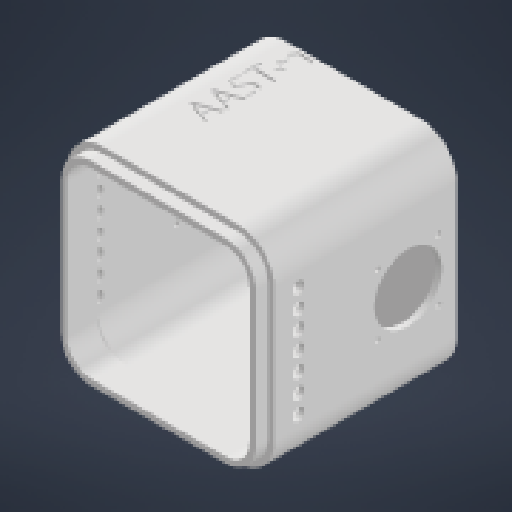
# Autodesk Inventor part: bottom case
Saved by Autodesk Inventor 2024 (Build 280153000, 153)
## iProperties
Created: 2023-06-18
Part Number: bottom case
Material: 일반
Document SubType Name: Modeling
Designer: 6gioc
Density: 1 g/cm^3
Appearance: 기본값
Author: 6gioc
Autodesk Inventor part; units mm, degrees
ref_plane "YZ Plane" through (0, 0, 0) normal (1, 0, 0) x (0, 1, 0)
ref_plane "XZ Plane" through (0, 0, 0) normal (0, 1, 0) x (-1, 0, 0)
ref_plane "XY Plane" through (0, 0, 0) normal (0, 0, 1) x (1, 0, 0)
sketch "스케치1" plane through (0, 0, 0) normal (0, 0, 1) x (1, 0, 0)
  line L0 (-30, 0) -> (-140, 0)
  line L1 (-170, -30) -> (-170, -140)
  line L2 (-140, -170) -> (-30, -170)
  line L3 (0, -140) -> (0, -30)
  arc A0 (-30, -170) -> (0, -140) centre (-30, -140) ccw
  arc A1 (-170, -140) -> (-140, -170) centre (-140, -140) ccw
  arc A2 (-140, 0) -> (-170, -30) centre (-140, -30) ccw
  arc A3 (0, -30) -> (-30, 0) centre (-30, -30) ccw
  point P0 (0, 0)
  point P1 (-170, -170)
  point P2 (-170, 0)
  point P3 (0, -170)
  dimension "d0" = 170
  dimension "d1" = 170
  dimension "d2" = 30
  dimension "d3" = 30
  dimension "d4" = 30
  constraints: 8 end point, 8 point on circle, 8 point on line, 8 tangent, 4 centre point, 2 parallel, 1 equal radius, 1 horizontal, 1 perpendicular
  measures "d0" distance of point (0, -170) point (-170, -170)
  measures "d1" distance of point (-170, -170) point (-170, 0)
  measures "d2" radius of A0
  measures "d3" radius of A1
  measures "d4" radius of A3
extrude "돌출1" add sketch "스케치1" along normal blind 150
shell "쉘1" thickness 5 removed faces 1 at (-66.6667, -113.3333, 150)
sketch "스케치2" plane through (0, 0, 150) normal (0, 0, 1) x (1, 0, 0)
  line L0 (-30, 0) -> (-140, 0)
  line L1 (-170, -30) -> (-170, -140)
  line L2 (-140, -170) -> (-30, -170)
  line L3 (0, -140) -> (0, -30)
  arc A0 (-30, -170) -> (0, -140) centre (-30, -140) ccw
  arc A1 (0, -30) -> (-30, 0) centre (-30, -30) ccw
  arc A2 (-140, 0) -> (-170, -30) centre (-140, -30) ccw
  arc A3 (-170, -140) -> (-140, -170) centre (-140, -140) ccw
  line L4 (-160, -30) -> (-160, -140)
  arc A4 (-160, -140) -> (-140, -160) centre (-140, -140) ccw
  line L5 (-140, -160) -> (-30, -160)
  arc A5 (-30, -160) -> (-10, -140) centre (-30, -140) ccw
  line L6 (-10, -140) -> (-10, -30)
  arc A6 (-10, -30) -> (-30, -10) centre (-30, -30) ccw
  line L7 (-30, -10) -> (-140, -10)
  arc A7 (-140, -10) -> (-160, -30) centre (-140, -30) ccw
  line L8 (-5, -140) -> (-5, -30)
  arc A8 (-5, -30) -> (-30, -5) centre (-30, -30) ccw
  line L9 (-30, -5) -> (-140, -5)
  arc A9 (-140, -5) -> (-165, -30) centre (-140, -30) ccw
  line L10 (-165, -30) -> (-165, -140)
  arc A10 (-165, -140) -> (-140, -165) centre (-140, -140) ccw
  line L11 (-140, -165) -> (-30, -165)
  arc A11 (-30, -165) -> (-5, -140) centre (-30, -140) ccw
  point P0 (0, 0)
  point P1 (-170, -170)
  point P2 (-170, 0)
  point P3 (0, -170)
  dimension "d8" = 170
  dimension "d9" = 170
  dimension "d10" = 30
  dimension "d11" = 10
  dimension "d17" = 5
  constraints: 24 end point, 24 point on circle, 12 centre point, 8 point on line, 8 tangent, 6 parallel, 3 equal radius, 3 perpendicular, 1 horizontal, 14 other
  measures "d8" distance of point (0, -170) point (-170, -170)
  measures "d9" distance of point (-170, -170) point (-170, 0)
  measures "d10" radius of A0
  measures "d11" radial gap between concentric circles of A2 A7
  measures "d17" radial gap between concentric circles of A0 A11
extrude "돌출2" add sketch "스케치2" against normal blind 20 contours A1 L3 A0 L2 A3 L1 A2 L0 | A11 L11 A10 L10 A9 L9 A8 L8
chamfer "모따기1" distance 5 angle 45 8 edges at (-85, -160, 130) (-15.8579, -154.1421, 130) (-10, -85, 130) (-15.8579, -15.8579, 130) (-85, -10, 130) (-154.1421, -15.8579, 130) (-160, -85, 130) (-154.1421, -154.1421, 130)
extrude "돌출3" add sketch "스케치2" along normal blind 10 contours A11 L11 A10 L10 A9 L9 A8 L8
sketch "스케치3" plane through (-140, 0, 0) normal (0, 1, 0) x (1, 0, 0)
  line L0 (23.785, -91.5699) -> (3.785, -84.2336)
  line L1 (3.785, -84.2336) -> (3.785, -81.9279)
  line L2 (3.785, -81.9279) -> (23.785, -74.6266)
  line L3 (23.785, -74.6266) -> (23.785, -77.107)
  line L4 (23.785, -77.107) -> (17.9509, -79.2205)
  line L5 (17.9509, -79.2205) -> (17.9509, -87.238)
  line L6 (17.9509, -87.238) -> (23.785, -89.2991)
  line L7 (23.785, -89.2991) -> (23.785, -91.5699)
  line L8 (6.9465, -83.2729) -> (15.9422, -86.5568)
  line L9 (15.9422, -86.5568) -> (15.9422, -79.9716)
  line L10 (15.9422, -79.9716) -> (6.9465, -83.2205)
  line L11 (6.9465, -83.2205) -> (6.9465, -83.2729)
  line L12 (23.785, -73.5262) -> (3.785, -66.1899)
  line L13 (3.785, -66.1899) -> (3.785, -63.8843)
  line L14 (3.785, -63.8843) -> (23.785, -56.583)
  line L15 (23.785, -56.583) -> (23.785, -59.0633)
  line L16 (23.785, -59.0633) -> (17.9509, -61.1768)
  line L17 (17.9509, -61.1768) -> (17.9509, -69.1943)
  line L18 (17.9509, -69.1943) -> (23.785, -71.2555)
  line L19 (23.785, -71.2555) -> (23.785, -73.5262)
  line L20 (6.9465, -65.2292) -> (15.9422, -68.5131)
  line L21 (15.9422, -68.5131) -> (15.9422, -61.9279)
  line L22 (15.9422, -61.9279) -> (6.9465, -65.1768)
  line L23 (6.9465, -65.1768) -> (6.9465, -65.2292)
  spline S0 degree 2 poles (24.1518, -49.1768) (24.1518, -52.4607) (22.8068, -54.8712) knots 0 0 0 1 1 1
  line L24 (22.8068, -54.8712) -> (20.8155, -54.8712)
  spline S1 degree 2 poles (20.8155, -54.8712) (22.1256, -52.321) (22.1256, -49.2817) knots 0 0 0 1 1 1
  spline S2 degree 2 poles (22.1256, -49.2817) (22.1256, -47.0284) (20.2042, -44.8624) (18.5098, -44.8624) knots 0 0 0 1 2 2 2
  spline S3 degree 2 poles (18.5098, -44.8624) (17.0251, -44.8624) (15.4356, -46.3821) (14.8417, -48.2511) knots 0 0 0 1 2 2 2
  line L25 (14.8417, -48.2511) -> (14.1605, -50.1899)
  spline S4 degree 2 poles (14.1605, -50.1899) (13.4094, -52.4083) (10.9465, -54.5742) (8.7631, -54.5742) knots 0 0 0 1 2 2 2
  spline S5 degree 2 poles (8.7631, -54.5742) (6.3526, -54.5742) (3.4531, -51.3952) (3.4531, -48.3559) knots 0 0 0 1 2 2 2
  spline S6 degree 2 poles (3.4531, -48.3559) (3.4531, -45.7533) (4.5535, -43.4825) knots 0 0 0 1 1 1
  line L26 (4.5535, -43.4825) -> (6.5622, -43.4825)
  spline S7 degree 2 poles (6.5622, -43.4825) (5.4443, -45.8755) (5.4443, -48.4432) knots 0 0 0 1 1 1
  spline S8 degree 2 poles (5.4443, -48.4432) (5.4443, -50.2598) (7.1212, -52.2511) (9.9858, -52.2511) (11.4705, -50.976) (12.0644, -49.2817) knots 0 0 0 1 2 3 4 4 4
  line L27 (12.0644, -49.2817) -> (12.6932, -47.3079)
  spline S9 degree 2 poles (12.6932, -47.3079) (13.5317, -44.8275) (15.9771, -42.4694) (18.3352, -42.4694) knots 0 0 0 1 2 2 2
  spline S10 degree 2 poles (18.3352, -42.4694) (21.0426, -42.4694) (24.1518, -45.7882) (24.1518, -49.1768) knots 0 0 0 1 2 2 2
  line L28 (23.785, -34.0677) -> (5.7762, -34.0677)
  line L29 (5.7762, -34.0677) -> (5.7762, -40.1812)
  line L30 (5.7762, -40.1812) -> (3.785, -40.1812)
  line L31 (3.785, -40.1812) -> (3.785, -25.631)
  line L32 (3.785, -25.631) -> (5.7762, -25.631)
  line L33 (5.7762, -25.631) -> (5.7762, -31.7445)
  line L34 (5.7762, -31.7445) -> (23.785, -31.7445)
  line L35 (23.785, -31.7445) -> (23.785, -34.0677)
  spline S11 degree 2 poles (9.9173, -17.3252) (11.1446, -16.9103) (12.5448, -14.4038) (12.5448, -13.1592) knots 0 0 0 1 2 2 2
  spline S12 degree 2 poles (12.5448, -13.1592) (12.5448, -11.6208) (10.9199, -8.9587) (9.416, -8.5438) knots 0 0 0 1 2 2 2
  spline S13 degree 2 poles (9.416, -8.5438) (9.8481, -6.7979) (11.8706, -3.7037) (12.804, -3.0469) knots 0 0 0 1 2 2 2
  spline S14 degree 2 poles (12.804, -3.0469) (13.8585, -2.3208) (15.2068, -2.3208) knots 0 0 0 1 1 1
  spline S15 degree 2 poles (15.2068, -2.3208) (16.123, -2.3208) (17.2811, -2.7703) knots 0 0 0 1 1 1
  spline S16 degree 2 poles (17.2811, -2.7703) (18.1973, -3.2197) (18.8369, -3.2197) knots 0 0 0 1 1 1
  spline S17 degree 2 poles (18.8369, -3.2197) (19.3036, -3.2197) (20.8594, -2.5801) knots 0 0 0 1 1 1
  spline S18 degree 2 poles (20.8594, -2.5801) (21.8447, -2.2863) (22.3114, -2.2863) knots 0 0 0 1 1 1
  spline S19 degree 2 poles (22.3114, -2.2863) (23.6943, -2.2863) (25.1117, -3.4617) knots 0 0 0 1 1 1
  spline S20 degree 2 poles (25.1117, -3.4617) (27.0651, -5.2422) (29.2258, -10.3243) (29.2258, -13.1074) knots 0 0 0 1 2 2 2
  spline S21 degree 2 poles (29.2258, -13.1074) (29.2258, -16.0114) (25.8378, -20.4367) (23.2103, -20.4367) knots 0 0 0 1 2 2 2
  spline S22 degree 2 poles (23.2103, -20.4367) (21.7755, -20.4367) (20.5482, -19.8144) knots 0 0 0 1 1 1
  spline S23 degree 2 poles (20.5482, -19.8144) (19.7185, -19.2958) (18.8715, -19.2958) knots 0 0 0 1 1 1
  spline S24 degree 2 poles (18.8715, -19.2958) (18.059, -19.2958) (17.2811, -19.6242) knots 0 0 0 1 1 1
  spline S25 degree 2 poles (17.2811, -19.6242) (15.2241, -20.4367) (14.4981, -20.4367) knots 0 0 0 1 1 1
  spline S26 degree 2 poles (14.4981, -20.4367) (12.5102, -20.4367) (11.0063, -19.0883) knots 0 0 0 1 1 1
  spline S27 degree 2 poles (11.0063, -19.0883) (10.384, -18.466) (9.9173, -17.3252) knots 0 0 0 1 1 1
  spline S28 degree 2 poles (19.7531, -19.6934) (19.7531, -21.8023) (18.3183, -23.5654) knots 0 0 0 1 1 1
  spline S29 degree 2 poles (18.3183, -23.5654) (16.97, -25.0348) (14.5672, -25.3805) knots 0 0 0 1 1 1
  spline S30 degree 2 poles (14.5672, -25.3805) (14.5672, -22.9604) (15.9328, -21.3528) knots 0 0 0 1 1 1
  spline S31 degree 2 poles (15.9328, -21.3528) (17.454, -19.6934) (19.7531, -19.6934) knots 0 0 0 1 1 1
  point P0 (140, 0)
  point P1 (3.4531, -92.1288)
  constraints: 1 other
extrude "돌출4" cut sketch "스케치3" against normal blind 2
sketch "스케치4" plane through (-140, -170, 0) normal (0, -1, 0) x (1, 0, 0)
  line L0 (-0.2518, 7.0228) -> (110.1783, 7.0228) construction
  line L1 (110.1783, 7.0228) -> (110.1783, 29.5331) construction
  line L2 (110.1783, 29.5331) -> (-0.2518, 29.5331) construction
  line L3 (-0.2518, 29.5331) -> (-0.2518, 7.0228) construction
  line L4 (82.8987, 6.8718) -> (109.9483, 6.8718) construction
  line L5 (109.9483, 6.8718) -> (109.9483, 3.7565) construction
  line L6 (109.9483, 3.7565) -> (82.8987, 3.7565) construction
  line L7 (82.8987, 3.7565) -> (82.8987, 6.8718) construction
  line L8 (6.2831, 27.4497) -> (5.0902, 27.4497)
  line L9 (5.0902, 27.4497) -> (1.5505, 34.3476)
  line L10 (1.5505, 34.3476) -> (1.5505, 27.4497)
  line L11 (1.5505, 27.4497) -> (0.5586, 27.4497)
  line L12 (0.5586, 27.4497) -> (0.5586, 35.4497)
  line L13 (0.5586, 35.4497) -> (2.0692, 35.4497)
  line L14 (2.0692, 35.4497) -> (5.2912, 29.1159)
  line L15 (5.2912, 29.1159) -> (5.2912, 35.4497)
  line L16 (5.2912, 35.4497) -> (6.2831, 35.4497)
  line L17 (6.2831, 35.4497) -> (6.2831, 27.4497)
  spline S0 degree 2 poles (13.5635, 34.5356) (14.0173, 34.004) (14.523, 32.4481) (14.523, 31.4497) knots 0 0 0 1 2 2 2
  spline S1 degree 2 poles (14.523, 31.4497) (14.523, 30.4773) (14.0303, 28.9019) (13.5635, 28.3703) knots 0 0 0 1 2 2 2
  spline S2 degree 2 poles (13.5635, 28.3703) (13.0708, 27.8128) (11.7677, 27.2812) (10.9833, 27.2812) knots 0 0 0 1 2 2 2
  spline S3 degree 2 poles (10.9833, 27.2812) (10.1729, 27.2812) (8.8763, 27.8322) (8.403, 28.3703) knots 0 0 0 1 2 2 2
  spline S4 degree 2 poles (8.403, 28.3703) (7.9427, 28.9019) (7.45, 30.4643) (7.45, 31.4497) knots 0 0 0 1 2 2 2
  spline S5 degree 2 poles (7.45, 31.4497) (7.45, 32.4546) (7.9492, 33.9846) (8.4095, 34.5356) knots 0 0 0 1 2 2 2
  spline S6 degree 2 poles (8.4095, 34.5356) (8.8763, 35.0672) (10.1794, 35.6183) (10.9833, 35.6183) knots 0 0 0 1 2 2 2
  spline S7 degree 2 poles (10.9833, 35.6183) (11.8001, 35.6183) (13.1097, 35.0478) (13.5635, 34.5356) knots 0 0 0 1 2 2 2
  spline S8 degree 2 poles (13.4144, 31.4497) (13.4144, 32.2407) (13.0708, 33.4659) (12.7596, 33.8679) knots 0 0 0 1 2 2 2
  spline S9 degree 2 poles (12.7596, 33.8679) (12.4419, 34.2828) (11.5473, 34.6977) (10.9897, 34.6977) knots 0 0 0 1 2 2 2
  spline S10 degree 2 poles (10.9897, 34.6977) (10.4128, 34.6977) (9.544, 34.2958) (9.2134, 33.8679) knots 0 0 0 1 2 2 2
  spline S11 degree 2 poles (9.2134, 33.8679) (8.8957, 33.4595) (8.5586, 32.2277) (8.5586, 31.4497) knots 0 0 0 1 2 2 2
  spline S12 degree 2 poles (8.5586, 31.4497) (8.5586, 29.8744) (9.8811, 28.2018) (10.9897, 28.2018) knots 0 0 0 1 2 2 2
  spline S13 degree 2 poles (10.9897, 28.2018) (12.0983, 28.2018) (13.4144, 29.8744) (13.4144, 31.4497) knots 0 0 0 1 2 2 2
  line L18 (17.557, 27.4497) -> (17.557, 34.5032)
  line L19 (17.557, 34.5032) -> (14.873, 34.5032)
  line L20 (14.873, 34.5032) -> (14.873, 35.4497)
  line L21 (14.873, 35.4497) -> (21.3042, 35.4497)
  line L22 (21.3042, 35.4497) -> (21.3042, 34.5032)
  line L23 (21.3042, 34.5032) -> (18.6202, 34.5032)
  line L24 (18.6202, 34.5032) -> (18.6202, 27.4497)
  line L25 (18.6202, 27.4497) -> (17.557, 27.4497)
  line L26 (30.335, 34.5032) -> (26.6137, 34.5032)
  line L27 (26.6137, 34.5032) -> (26.6137, 32.2471)
  line L28 (26.6137, 32.2471) -> (30.1794, 32.2471)
  line L29 (30.1794, 32.2471) -> (30.1794, 31.3006)
  line L30 (30.1794, 31.3006) -> (26.6137, 31.3006)
  line L31 (26.6137, 31.3006) -> (26.6137, 27.4497)
  line L32 (26.6137, 27.4497) -> (25.5505, 27.4497)
  line L33 (25.5505, 27.4497) -> (25.5505, 35.4497)
  line L34 (25.5505, 35.4497) -> (30.335, 35.4497)
  line L35 (30.335, 35.4497) -> (30.335, 34.5032)
  spline S14 degree 2 poles (36.9476, 34.5356) (37.4014, 34.004) (37.9071, 32.4481) (37.9071, 31.4497) knots 0 0 0 1 2 2 2
  spline S15 degree 2 poles (37.9071, 31.4497) (37.9071, 30.4773) (37.4144, 28.9019) (36.9476, 28.3703) knots 0 0 0 1 2 2 2
  spline S16 degree 2 poles (36.9476, 28.3703) (36.4549, 27.8128) (35.1518, 27.2812) (34.3674, 27.2812) knots 0 0 0 1 2 2 2
  spline S17 degree 2 poles (34.3674, 27.2812) (33.557, 27.2812) (32.2604, 27.8322) (31.7871, 28.3703) knots 0 0 0 1 2 2 2
  spline S18 degree 2 poles (31.7871, 28.3703) (31.3269, 28.9019) (30.8341, 30.4643) (30.8341, 31.4497) knots 0 0 0 1 2 2 2
  spline S19 degree 2 poles (30.8341, 31.4497) (30.8341, 32.4546) (31.3333, 33.9846) (31.7936, 34.5356) knots 0 0 0 1 2 2 2
  spline S20 degree 2 poles (31.7936, 34.5356) (32.2604, 35.0672) (33.5635, 35.6183) (34.3674, 35.6183) knots 0 0 0 1 2 2 2
  spline S21 degree 2 poles (34.3674, 35.6183) (35.1842, 35.6183) (36.4938, 35.0478) (36.9476, 34.5356) knots 0 0 0 1 2 2 2
  spline S22 degree 2 poles (36.7985, 31.4497) (36.7985, 32.2407) (36.4549, 33.4659) (36.1437, 33.8679) knots 0 0 0 1 2 2 2
  spline S23 degree 2 poles (36.1437, 33.8679) (35.826, 34.2828) (34.9314, 34.6977) (34.3739, 34.6977) knots 0 0 0 1 2 2 2
  spline S24 degree 2 poles (34.3739, 34.6977) (33.7969, 34.6977) (32.9281, 34.2958) (32.5975, 33.8679) knots 0 0 0 1 2 2 2
  spline S25 degree 2 poles (32.5975, 33.8679) (32.2799, 33.4595) (31.9427, 32.2277) (31.9427, 31.4497) knots 0 0 0 1 2 2 2
  spline S26 degree 2 poles (31.9427, 31.4497) (31.9427, 29.8744) (33.2653, 28.2018) (34.3739, 28.2018) knots 0 0 0 1 2 2 2
  spline S27 degree 2 poles (34.3739, 28.2018) (35.4824, 28.2018) (36.7985, 29.8744) (36.7985, 31.4497) knots 0 0 0 1 2 2 2
  line L36 (45.2653, 27.4497) -> (43.8844, 27.4497)
  line L37 (43.8844, 27.4497) -> (41.356, 30.6329)
  line L38 (41.356, 30.6329) -> (40.1372, 30.6329)
  line L39 (40.1372, 30.6329) -> (40.1372, 27.4497)
  line L40 (40.1372, 27.4497) -> (39.074, 27.4497)
  line L41 (39.074, 27.4497) -> (39.074, 35.4497)
  line L42 (39.074, 35.4497) -> (41.1356, 35.4497)
  spline S28 degree 2 poles (41.1356, 35.4497) (41.8228, 35.4497) (42.7499, 35.3006) (43.1713, 35.0283) knots 0 0 0 1 2 2 2
  spline S29 degree 2 poles (43.1713, 35.0283) (43.5927, 34.756) (44.0789, 33.9068) (44.0789, 33.2779) knots 0 0 0 1 2 2 2
  spline S30 degree 2 poles (44.0789, 33.2779) (44.0789, 32.4027) (43.1842, 31.2163) (42.4192, 30.9311) knots 0 0 0 1 2 2 2
  line L43 (42.4192, 30.9311) -> (45.2653, 27.4497)
  spline S31 degree 2 poles (42.9703, 33.1937) (42.9703, 33.5437) (42.7239, 34.0818) (42.4646, 34.2569) knots 0 0 0 1 2 2 2
  spline S32 degree 2 poles (42.4646, 34.2569) (42.2377, 34.406) (41.6348, 34.5291) (41.194, 34.5291) knots 0 0 0 1 2 2 2
  line L44 (41.194, 34.5291) -> (40.1372, 34.5291)
  line L45 (40.1372, 34.5291) -> (40.1372, 31.521)
  line L46 (40.1372, 31.521) -> (41.0708, 31.521)
  spline S33 degree 2 poles (41.0708, 31.521) (41.5311, 31.521) (42.2636, 31.6831) (42.5165, 31.936) knots 0 0 0 1 2 2 2
  spline S34 degree 2 poles (42.5165, 31.936) (42.7499, 32.1564) (42.9703, 32.7787) (42.9703, 33.1937) knots 0 0 0 1 2 2 2
  line L47 (7.4176, 14.2779) -> (6.3544, 14.2779)
  line L48 (6.3544, 14.2779) -> (6.3544, 21.1694)
  line L49 (6.3544, 21.1694) -> (4.2669, 16.4822)
  line L50 (4.2669, 16.4822) -> (3.6186, 16.4822)
  line L51 (3.6186, 16.4822) -> (1.5505, 21.1694)
  line L52 (1.5505, 21.1694) -> (1.5505, 14.2779)
  line L53 (1.5505, 14.2779) -> (0.5586, 14.2779)
  line L54 (0.5586, 14.2779) -> (0.5586, 22.2779)
  line L55 (0.5586, 22.2779) -> (2.0108, 22.2779)
  line L56 (2.0108, 22.2779) -> (4.0076, 17.8241)
  line L57 (4.0076, 17.8241) -> (5.9395, 22.2779)
  line L58 (5.9395, 22.2779) -> (7.4176, 22.2779)
  line L59 (7.4176, 22.2779) -> (7.4176, 14.2779)
  line L60 (11.826, 14.2779) -> (8.7272, 14.2779)
  line L61 (8.7272, 14.2779) -> (8.7272, 15.0948)
  line L62 (8.7272, 15.0948) -> (9.745, 15.0948)
  line L63 (9.745, 15.0948) -> (9.745, 21.4611)
  line L64 (9.745, 21.4611) -> (8.7272, 21.4611)
  line L65 (8.7272, 21.4611) -> (8.7272, 22.2779)
  line L66 (8.7272, 22.2779) -> (11.826, 22.2779)
  line L67 (11.826, 22.2779) -> (11.826, 21.4611)
  line L68 (11.826, 21.4611) -> (10.8082, 21.4611)
  line L69 (10.8082, 21.4611) -> (10.8082, 15.0948)
  line L70 (10.8082, 15.0948) -> (11.826, 15.0948)
  line L71 (11.826, 15.0948) -> (11.826, 14.2779)
  line L72 (17.7774, 14.2779) -> (13.1421, 14.2779)
  line L73 (13.1421, 14.2779) -> (13.1421, 22.2779)
  line L74 (13.1421, 22.2779) -> (14.2053, 22.2779)
  line L75 (14.2053, 22.2779) -> (14.2053, 15.2245)
  line L76 (14.2053, 15.2245) -> (17.7774, 15.2245)
  line L77 (17.7774, 15.2245) -> (17.7774, 14.2779)
  line L78 (21.4014, 14.2779) -> (18.3025, 14.2779)
  line L79 (18.3025, 14.2779) -> (18.3025, 15.0948)
  line L80 (18.3025, 15.0948) -> (19.3204, 15.0948)
  line L81 (19.3204, 15.0948) -> (19.3204, 21.4611)
  line L82 (19.3204, 21.4611) -> (18.3025, 21.4611)
  line L83 (18.3025, 21.4611) -> (18.3025, 22.2779)
  line L84 (18.3025, 22.2779) -> (21.4014, 22.2779)
  line L85 (21.4014, 22.2779) -> (21.4014, 21.4611)
  line L86 (21.4014, 21.4611) -> (20.3836, 21.4611)
  line L87 (20.3836, 21.4611) -> (20.3836, 15.0948)
  line L88 (20.3836, 15.0948) -> (21.4014, 15.0948)
  line L89 (21.4014, 15.0948) -> (21.4014, 14.2779)
  line L90 (24.5846, 14.2779) -> (24.5846, 21.3314)
  line L91 (24.5846, 21.3314) -> (21.9006, 21.3314)
  line L92 (21.9006, 21.3314) -> (21.9006, 22.2779)
  line L93 (21.9006, 22.2779) -> (28.3317, 22.2779)
  line L94 (28.3317, 22.2779) -> (28.3317, 21.3314)
  line L95 (28.3317, 21.3314) -> (25.6478, 21.3314)
  line L96 (25.6478, 21.3314) -> (25.6478, 14.2779)
  line L97 (25.6478, 14.2779) -> (24.5846, 14.2779)
  line L98 (28.2799, 14.2779) -> (30.9768, 22.2779)
  line L99 (30.9768, 22.2779) -> (32.2863, 22.2779)
  line L100 (32.2863, 22.2779) -> (34.9833, 14.2779)
  line L101 (34.9833, 14.2779) -> (33.8617, 14.2779)
  line L102 (33.8617, 14.2779) -> (33.1356, 16.5146)
  line L103 (33.1356, 16.5146) -> (30.0821, 16.5146)
  line L104 (30.0821, 16.5146) -> (29.356, 14.2779)
  line L105 (29.356, 14.2779) -> (28.2799, 14.2779)
  line L106 (32.8439, 17.4222) -> (31.6056, 21.1888)
  line L107 (31.6056, 21.1888) -> (30.3739, 17.4222)
  line L108 (30.3739, 17.4222) -> (32.8439, 17.4222)
  line L109 (41.933, 14.2779) -> (40.5521, 14.2779)
  line L110 (40.5521, 14.2779) -> (38.0238, 17.4611)
  line L111 (38.0238, 17.4611) -> (36.805, 17.4611)
  line L112 (36.805, 17.4611) -> (36.805, 14.2779)
  line L113 (36.805, 14.2779) -> (35.7418, 14.2779)
  line L114 (35.7418, 14.2779) -> (35.7418, 22.2779)
  line L115 (35.7418, 22.2779) -> (37.8034, 22.2779)
  spline S35 degree 2 poles (37.8034, 22.2779) (38.4905, 22.2779) (39.4176, 22.1288) (39.839, 21.8565) knots 0 0 0 1 2 2 2
  spline S36 degree 2 poles (39.839, 21.8565) (40.2604, 21.5843) (40.7466, 20.735) (40.7466, 20.1061) knots 0 0 0 1 2 2 2
  spline S37 degree 2 poles (40.7466, 20.1061) (40.7466, 19.2309) (39.852, 18.0446) (39.087, 17.7593) knots 0 0 0 1 2 2 2
  line L116 (39.087, 17.7593) -> (41.933, 14.2779)
  spline S38 degree 2 poles (39.638, 20.0219) (39.638, 20.3719) (39.3917, 20.91) (39.1324, 21.0851) knots 0 0 0 1 2 2 2
  spline S39 degree 2 poles (39.1324, 21.0851) (38.9055, 21.2342) (38.3025, 21.3574) (37.8617, 21.3574) knots 0 0 0 1 2 2 2
  line L117 (37.8617, 21.3574) -> (36.805, 21.3574)
  line L118 (36.805, 21.3574) -> (36.805, 18.3493)
  line L119 (36.805, 18.3493) -> (37.7385, 18.3493)
  spline S40 degree 2 poles (37.7385, 18.3493) (38.1988, 18.3493) (38.9314, 18.5113) (39.1842, 18.7642) knots 0 0 0 1 2 2 2
  spline S41 degree 2 poles (39.1842, 18.7642) (39.4176, 18.9846) (39.638, 19.607) (39.638, 20.0219) knots 0 0 0 1 2 2 2
  line L120 (48.1696, 22.2779) -> (45.4662, 17.8176)
  line L121 (45.4662, 17.8176) -> (45.4662, 14.2779)
  line L122 (45.4662, 14.2779) -> (44.403, 14.2779)
  line L123 (44.403, 14.2779) -> (44.403, 17.7074)
  line L124 (44.403, 17.7074) -> (41.6996, 22.2779)
  line L125 (41.6996, 22.2779) -> (42.8795, 22.2779)
  line L126 (42.8795, 22.2779) -> (44.9411, 18.7577)
  line L127 (44.9411, 18.7577) -> (47.0416, 22.2779)
  line L128 (47.0416, 22.2779) -> (48.1696, 22.2779)
  spline S42 degree 2 poles (5.6153, 6.6945) (5.6153, 6.1758) (5.2458, 5.2423) (4.9152, 4.9181) knots 0 0 0 1 2 2 2
  spline S43 degree 2 poles (4.9152, 4.9181) (4.5003, 4.5097) (3.3787, 4.0883) (2.523, 4.0883) knots 0 0 0 1 2 2 2
  line L129 (2.523, 4.0883) -> (1.6218, 4.0883)
  line L130 (1.6218, 4.0883) -> (1.6218, 1.1062)
  line L131 (1.6218, 1.1062) -> (0.5586, 1.1062)
  line L132 (0.5586, 1.1062) -> (0.5586, 9.1062)
  line L133 (0.5586, 9.1062) -> (2.5683, 9.1062)
  spline S44 degree 2 poles (2.5683, 9.1062) (3.2815, 9.1062) (4.2799, 8.8728) (4.6623, 8.607) knots 0 0 0 1 2 2 2
  spline S45 degree 2 poles (4.6623, 8.607) (5.1097, 8.3023) (5.6153, 7.3622) (5.6153, 6.6945) knots 0 0 0 1 2 2 2
  spline S46 degree 2 poles (4.5068, 6.6621) (4.5068, 7.077) (4.2215, 7.6864) (3.9298, 7.8809) knots 0 0 0 1 2 2 2
  spline S47 degree 2 poles (3.9298, 7.8809) (3.6769, 8.0494) (3.0027, 8.1856) (2.5035, 8.1856) knots 0 0 0 1 2 2 2
  line L134 (2.5035, 8.1856) -> (1.6218, 8.1856)
  line L135 (1.6218, 8.1856) -> (1.6218, 4.9959)
  line L136 (1.6218, 4.9959) -> (2.3479, 4.9959)
  spline S48 degree 2 poles (2.3479, 4.9959) (2.9962, 4.9959) (3.7936, 5.2034) (4.0529, 5.4757) knots 0 0 0 1 2 2 2
  spline S49 degree 2 poles (4.0529, 5.4757) (4.2928, 5.7156) (4.5068, 6.2796) (4.5068, 6.6621) knots 0 0 0 1 2 2 2
  line L137 (6.6267, 1.1062) -> (6.6267, 9.1062)
  line L138 (6.6267, 9.1062) -> (11.6316, 9.1062)
  line L139 (11.6316, 9.1062) -> (11.6316, 8.1596)
  line L140 (11.6316, 8.1596) -> (7.6899, 8.1596)
  line L141 (7.6899, 8.1596) -> (7.6899, 5.9684)
  line L142 (7.6899, 5.9684) -> (11.3658, 5.9684)
  line L143 (11.3658, 5.9684) -> (11.3658, 5.0219)
  line L144 (11.3658, 5.0219) -> (7.6899, 5.0219)
  line L145 (7.6899, 5.0219) -> (7.6899, 2.0527)
  line L146 (7.6899, 2.0527) -> (11.6316, 2.0527)
  line L147 (11.6316, 2.0527) -> (11.6316, 1.1062)
  line L148 (11.6316, 1.1062) -> (6.6267, 1.1062)
  line L149 (18.9897, 1.1062) -> (17.6089, 1.1062)
  line L150 (17.6089, 1.1062) -> (15.0805, 4.2893)
  line L151 (15.0805, 4.2893) -> (13.8617, 4.2893)
  line L152 (13.8617, 4.2893) -> (13.8617, 1.1062)
  line L153 (13.8617, 1.1062) -> (12.7985, 1.1062)
  line L154 (12.7985, 1.1062) -> (12.7985, 9.1062)
  line L155 (12.7985, 9.1062) -> (14.8601, 9.1062)
  spline S50 degree 2 poles (14.8601, 9.1062) (15.5473, 9.1062) (16.4743, 8.957) (16.8957, 8.6848) knots 0 0 0 1 2 2 2
  spline S51 degree 2 poles (16.8957, 8.6848) (17.3171, 8.4125) (17.8034, 7.5632) (17.8034, 6.9344) knots 0 0 0 1 2 2 2
  spline S52 degree 2 poles (17.8034, 6.9344) (17.8034, 6.0591) (16.9087, 4.8728) (16.1437, 4.5875) knots 0 0 0 1 2 2 2
  line L156 (16.1437, 4.5875) -> (18.9897, 1.1062)
  spline S53 degree 2 poles (16.6948, 6.8501) (16.6948, 7.2002) (16.4484, 7.7382) (16.1891, 7.9133) knots 0 0 0 1 2 2 2
  spline S54 degree 2 poles (16.1891, 7.9133) (15.9622, 8.0624) (15.3593, 8.1856) (14.9184, 8.1856) knots 0 0 0 1 2 2 2
  line L157 (14.9184, 8.1856) -> (13.8617, 8.1856)
  line L158 (13.8617, 8.1856) -> (13.8617, 5.1775)
  line L159 (13.8617, 5.1775) -> (14.7952, 5.1775)
  spline S55 degree 2 poles (14.7952, 5.1775) (15.2555, 5.1775) (15.9881, 5.3395) (16.241, 5.5924) knots 0 0 0 1 2 2 2
  spline S56 degree 2 poles (16.241, 5.5924) (16.4743, 5.8128) (16.6948, 6.4352) (16.6948, 6.8501) knots 0 0 0 1 2 2 2
  spline S57 degree 2 poles (24.6818, 6.6945) (24.6818, 6.1758) (24.3123, 5.2423) (23.9816, 4.9181) knots 0 0 0 1 2 2 2
  spline S58 degree 2 poles (23.9816, 4.9181) (23.5667, 4.5097) (22.4452, 4.0883) (21.5894, 4.0883) knots 0 0 0 1 2 2 2
  line L160 (21.5894, 4.0883) -> (20.6883, 4.0883)
  line L161 (20.6883, 4.0883) -> (20.6883, 1.1062)
  line L162 (20.6883, 1.1062) -> (19.6251, 1.1062)
  line L163 (19.6251, 1.1062) -> (19.6251, 9.1062)
  line L164 (19.6251, 9.1062) -> (21.6348, 9.1062)
  spline S59 degree 2 poles (21.6348, 9.1062) (22.3479, 9.1062) (23.3463, 8.8728) (23.7288, 8.607) knots 0 0 0 1 2 2 2
  spline S60 degree 2 poles (23.7288, 8.607) (24.1761, 8.3023) (24.6818, 7.3622) (24.6818, 6.6945) knots 0 0 0 1 2 2 2
  spline S61 degree 2 poles (23.5732, 6.6621) (23.5732, 7.077) (23.288, 7.6864) (22.9962, 7.8809) knots 0 0 0 1 2 2 2
  spline S62 degree 2 poles (22.9962, 7.8809) (22.7434, 8.0494) (22.0692, 8.1856) (21.57, 8.1856) knots 0 0 0 1 2 2 2
  line L165 (21.57, 8.1856) -> (20.6883, 8.1856)
  line L166 (20.6883, 8.1856) -> (20.6883, 4.9959)
  line L167 (20.6883, 4.9959) -> (21.4144, 4.9959)
  spline S63 degree 2 poles (21.4144, 4.9959) (22.0627, 4.9959) (22.8601, 5.2034) (23.1194, 5.4757) knots 0 0 0 1 2 2 2
  spline S64 degree 2 poles (23.1194, 5.4757) (23.3593, 5.7156) (23.5732, 6.2796) (23.5732, 6.6621) knots 0 0 0 1 2 2 2
  spline S65 degree 2 poles (31.3528, 8.1921) (31.8066, 7.6604) (32.3123, 6.1045) (32.3123, 5.1062) knots 0 0 0 1 2 2 2
  spline S66 degree 2 poles (32.3123, 5.1062) (32.3123, 4.1337) (31.8196, 2.5583) (31.3528, 2.0267) knots 0 0 0 1 2 2 2
  spline S67 degree 2 poles (31.3528, 2.0267) (30.8601, 1.4692) (29.557, 0.9376) (28.7726, 0.9376) knots 0 0 0 1 2 2 2
  spline S68 degree 2 poles (28.7726, 0.9376) (27.9622, 0.9376) (26.6656, 1.4886) (26.1923, 2.0267) knots 0 0 0 1 2 2 2
  spline S69 degree 2 poles (26.1923, 2.0267) (25.732, 2.5583) (25.2393, 4.1207) (25.2393, 5.1062) knots 0 0 0 1 2 2 2
  spline S70 degree 2 poles (25.2393, 5.1062) (25.2393, 6.111) (25.7385, 7.641) (26.1988, 8.1921) knots 0 0 0 1 2 2 2
  spline S71 degree 2 poles (26.1988, 8.1921) (26.6656, 8.7237) (27.9687, 9.2747) (28.7726, 9.2747) knots 0 0 0 1 2 2 2
  spline S72 degree 2 poles (28.7726, 9.2747) (29.5894, 9.2747) (30.899, 8.7042) (31.3528, 8.1921) knots 0 0 0 1 2 2 2
  spline S73 degree 2 poles (31.2037, 5.1062) (31.2037, 5.8971) (30.8601, 7.1224) (30.5489, 7.5243) knots 0 0 0 1 2 2 2
  spline S74 degree 2 poles (30.5489, 7.5243) (30.2312, 7.9392) (29.3366, 8.3541) (28.779, 8.3541) knots 0 0 0 1 2 2 2
  spline S75 degree 2 poles (28.779, 8.3541) (28.2021, 8.3541) (27.3333, 7.9522) (27.0027, 7.5243) knots 0 0 0 1 2 2 2
  spline S76 degree 2 poles (27.0027, 7.5243) (26.685, 7.1159) (26.3479, 5.8841) (26.3479, 5.1062) knots 0 0 0 1 2 2 2
  spline S77 degree 2 poles (26.3479, 5.1062) (26.3479, 3.5308) (27.6705, 1.8582) (28.779, 1.8582) knots 0 0 0 1 2 2 2
  spline S78 degree 2 poles (28.779, 1.8582) (29.8876, 1.8582) (31.2037, 3.5308) (31.2037, 5.1062) knots 0 0 0 1 2 2 2
  spline S79 degree 2 poles (35.7093, 0.9635) (34.8406, 0.9635) (33.6218, 1.3266) (33.0837, 1.5859) knots 0 0 0 1 2 2 2
  line L168 (33.0837, 1.5859) -> (33.0837, 2.9214)
  line L169 (33.0837, 2.9214) -> (33.1615, 2.9214)
  spline S80 degree 2 poles (33.1615, 2.9214) (33.6867, 2.4287) (35.0157, 1.8841) (35.6316, 1.8841) knots 0 0 0 1 2 2 2
  spline S81 degree 2 poles (35.6316, 1.8841) (36.5132, 1.8841) (37.4144, 2.6167) (37.4144, 3.2196) knots 0 0 0 1 2 2 2
  spline S82 degree 2 poles (37.4144, 3.2196) (37.4144, 3.6993) (36.9411, 4.2958) (36.429, 4.4449) knots 0 0 0 1 2 2 2
  spline S83 degree 2 poles (36.429, 4.4449) (36.0594, 4.5486) (35.4435, 4.6912) (34.9833, 4.8079) knots 0 0 0 1 2 2 2
  spline S84 degree 2 poles (34.9833, 4.8079) (34.5683, 4.9181) (33.9136, 5.2488) (33.6607, 5.5146) knots 0 0 0 1 2 2 2
  spline S85 degree 2 poles (33.6607, 5.5146) (33.4144, 5.7804) (33.1421, 6.4935) (33.1421, 6.9603) knots 0 0 0 1 2 2 2
  spline S86 degree 2 poles (33.1421, 6.9603) (33.1421, 7.9327) (34.6591, 9.2488) (35.8325, 9.2488) knots 0 0 0 1 2 2 2
  spline S87 degree 2 poles (35.8325, 9.2488) (36.5068, 9.2488) (37.6996, 8.983) (38.2118, 8.7301) knots 0 0 0 1 2 2 2
  line L170 (38.2118, 8.7301) -> (38.2118, 7.4595)
  line L171 (38.2118, 7.4595) -> (38.134, 7.4595)
  spline S88 degree 2 poles (38.134, 7.4595) (37.7515, 7.8096) (36.5586, 8.3282) (35.9038, 8.3282) knots 0 0 0 1 2 2 2
  spline S89 degree 2 poles (35.9038, 8.3282) (35.1648, 8.3282) (34.2507, 7.6345) (34.2507, 7.0705) knots 0 0 0 1 2 2 2
  spline S90 degree 2 poles (34.2507, 7.0705) (34.2507, 6.5648) (34.7888, 5.9619) (35.2944, 5.8258) knots 0 0 0 1 2 2 2
  spline S91 degree 2 poles (35.2944, 5.8258) (35.6316, 5.735) (36.6105, 5.5016) (36.9346, 5.4044) knots 0 0 0 1 2 2 2
  spline S92 degree 2 poles (36.9346, 5.4044) (37.758, 5.1515) (38.523, 4.1337) (38.523, 3.3882) knots 0 0 0 1 2 2 2
  spline S93 degree 2 poles (38.523, 3.3882) (38.523, 2.9149) (38.1405, 2.0073) (37.7969, 1.6896) knots 0 0 0 1 2 2 2
  spline S94 degree 2 poles (37.7969, 1.6896) (37.4144, 1.3395) (36.4419, 0.9635) (35.7093, 0.9635) knots 0 0 0 1 2 2 2
  line L172 (39.6056, 1.1062) -> (39.6056, 9.1062)
  line L173 (39.6056, 9.1062) -> (44.6105, 9.1062)
  line L174 (44.6105, 9.1062) -> (44.6105, 8.1596)
  line L175 (44.6105, 8.1596) -> (40.6688, 8.1596)
  line L176 (40.6688, 8.1596) -> (40.6688, 5.9684)
  line L177 (40.6688, 5.9684) -> (44.3447, 5.9684)
  line L178 (44.3447, 5.9684) -> (44.3447, 5.0219)
  line L179 (44.3447, 5.0219) -> (40.6688, 5.0219)
  line L180 (40.6688, 5.0219) -> (40.6688, 2.0527)
  line L181 (40.6688, 2.0527) -> (44.6105, 2.0527)
  line L182 (44.6105, 2.0527) -> (44.6105, 1.1062)
  line L183 (44.6105, 1.1062) -> (39.6056, 1.1062)
  spline S95 degree 2 poles (85.2171, 0.5394) (84.5547, 0.5394) (83.6253, 0.8163) (83.2151, 1.014) knots 0 0 0 1 2 2 2
  line L184 (83.2151, 1.014) -> (83.2151, 2.0323)
  line L185 (83.2151, 2.0323) -> (83.2744, 2.0323)
  spline S96 degree 2 poles (83.2744, 2.0323) (83.6748, 1.6566) (84.6881, 1.2414) (85.1578, 1.2414) knots 0 0 0 1 2 2 2
  spline S97 degree 2 poles (85.1578, 1.2414) (85.83, 1.2414) (86.5172, 1.8) (86.5172, 2.2597) knots 0 0 0 1 2 2 2
  spline S98 degree 2 poles (86.5172, 2.2597) (86.5172, 2.6255) (86.1563, 3.0803) (85.7658, 3.194) knots 0 0 0 1 2 2 2
  spline S99 degree 2 poles (85.7658, 3.194) (85.484, 3.2731) (85.0144, 3.3818) (84.6634, 3.4708) knots 0 0 0 1 2 2 2
  spline S100 degree 2 poles (84.6634, 3.4708) (84.3471, 3.5548) (83.8478, 3.8069) (83.655, 4.0096) knots 0 0 0 1 2 2 2
  spline S101 degree 2 poles (83.655, 4.0096) (83.4672, 4.2123) (83.2595, 4.756) (83.2595, 5.112) knots 0 0 0 1 2 2 2
  spline S102 degree 2 poles (83.2595, 5.112) (83.2595, 5.8535) (84.4163, 6.8569) (85.311, 6.8569) knots 0 0 0 1 2 2 2
  spline S103 degree 2 poles (85.311, 6.8569) (85.8251, 6.8569) (86.7347, 6.6543) (87.1252, 6.4615) knots 0 0 0 1 2 2 2
  line L186 (87.1252, 6.4615) -> (87.1252, 5.4926)
  line L187 (87.1252, 5.4926) -> (87.0659, 5.4926)
  spline S104 degree 2 poles (87.0659, 5.4926) (86.7742, 5.7595) (85.8646, 6.155) (85.3654, 6.155) knots 0 0 0 1 2 2 2
  spline S105 degree 2 poles (85.3654, 6.155) (84.8018, 6.155) (84.1048, 5.6261) (84.1048, 5.196) knots 0 0 0 1 2 2 2
  spline S106 degree 2 poles (84.1048, 5.196) (84.1048, 4.8104) (84.5151, 4.3507) (84.9007, 4.2469) knots 0 0 0 1 2 2 2
  spline S107 degree 2 poles (84.9007, 4.2469) (85.1578, 4.1777) (85.9042, 3.9997) (86.1514, 3.9256) knots 0 0 0 1 2 2 2
  spline S108 degree 2 poles (86.1514, 3.9256) (86.7792, 3.7328) (87.3625, 2.9567) (87.3625, 2.3882) knots 0 0 0 1 2 2 2
  spline S109 degree 2 poles (87.3625, 2.3882) (87.3625, 2.0274) (87.0708, 1.3353) (86.8088, 1.0931) knots 0 0 0 1 2 2 2
  spline S110 degree 2 poles (86.8088, 1.0931) (86.5172, 0.8261) (85.7757, 0.5394) (85.2171, 0.5394) knots 0 0 0 1 2 2 2
  line L188 (92.5529, 0.6482) -> (91.6433, 0.6482)
  line L189 (91.6433, 0.6482) -> (88.9443, 5.9078)
  line L190 (88.9443, 5.9078) -> (88.9443, 0.6482)
  line L191 (88.9443, 0.6482) -> (88.188, 0.6482)
  line L192 (88.188, 0.6482) -> (88.188, 6.7482)
  line L193 (88.188, 6.7482) -> (89.3398, 6.7482)
  line L194 (89.3398, 6.7482) -> (91.7966, 1.9186)
  line L195 (91.7966, 1.9186) -> (91.7966, 6.7482)
  line L196 (91.7966, 6.7482) -> (92.5529, 6.7482)
  line L197 (92.5529, 6.7482) -> (92.5529, 0.6482)
  line L198 (95.8501, 2.9468) -> (93.5416, 2.9468)
  line L199 (93.5416, 2.9468) -> (93.5416, 3.6883)
  line L200 (93.5416, 3.6883) -> (95.8501, 3.6883)
  line L201 (95.8501, 3.6883) -> (95.8501, 2.9468)
  spline S111 degree 2 poles (100.4572, 3.6982) (100.4572, 2.057) (99.5031, 0.5197) (98.5095, 0.5197) knots 0 0 0 1 2 2 2
  spline S112 degree 2 poles (98.5095, 0.5197) (97.5011, 0.5197) (96.5569, 2.0867) (96.5569, 3.6932) knots 0 0 0 1 2 2 2
  spline S113 degree 2 poles (96.5569, 3.6932) (96.5569, 5.3443) (97.511, 6.8718) (98.5095, 6.8718) knots 0 0 0 1 2 2 2
  spline S114 degree 2 poles (98.5095, 6.8718) (99.513, 6.8718) (100.4572, 5.2899) (100.4572, 3.6982) knots 0 0 0 1 2 2 2
  spline S115 degree 2 poles (99.4092, 1.8395) (99.5279, 2.1411) (99.6267, 3.0704) (99.6267, 3.6982) knots 0 0 0 1 2 2 2
  spline S116 degree 2 poles (99.6267, 3.6982) (99.6267, 4.326) (99.5279, 5.2504) (99.4043, 5.5618) knots 0 0 0 1 2 2 2
  spline S117 degree 2 poles (99.4043, 5.5618) (99.2807, 5.8732) (98.8506, 6.1945) (98.5095, 6.1945) knots 0 0 0 1 2 2 2
  spline S118 degree 2 poles (98.5095, 6.1945) (98.1685, 6.1945) (97.7285, 5.8732) (97.6, 5.5519) knots 0 0 0 1 2 2 2
  spline S119 degree 2 poles (97.6, 5.5519) (97.4764, 5.2405) (97.3874, 4.2914) (97.3874, 3.6932) knots 0 0 0 1 2 2 2
  spline S120 degree 2 poles (97.3874, 3.6932) (97.3874, 3.0506) (97.4665, 2.1905) (97.595, 1.8543) knots 0 0 0 1 2 2 2
  spline S121 degree 2 poles (97.595, 1.8543) (97.7137, 1.538) (98.1536, 1.1969) (98.5095, 1.1969) knots 0 0 0 1 2 2 2
  spline S122 degree 2 poles (98.5095, 1.1969) (98.8457, 1.1969) (99.2856, 1.5182) (99.4092, 1.8395) knots 0 0 0 1 2 2 2
  spline S123 degree 2 poles (105.0347, 3.6982) (105.0347, 2.057) (104.0806, 0.5197) (103.087, 0.5197) knots 0 0 0 1 2 2 2
  spline S124 degree 2 poles (103.087, 0.5197) (102.0786, 0.5197) (101.1344, 2.0867) (101.1344, 3.6932) knots 0 0 0 1 2 2 2
  spline S125 degree 2 poles (101.1344, 3.6932) (101.1344, 5.3443) (102.0885, 6.8718) (103.087, 6.8718) knots 0 0 0 1 2 2 2
  spline S126 degree 2 poles (103.087, 6.8718) (104.0905, 6.8718) (105.0347, 5.2899) (105.0347, 3.6982) knots 0 0 0 1 2 2 2
  spline S127 degree 2 poles (103.9867, 1.8395) (104.1053, 2.1411) (104.2042, 3.0704) (104.2042, 3.6982) knots 0 0 0 1 2 2 2
  spline S128 degree 2 poles (104.2042, 3.6982) (104.2042, 4.326) (104.1053, 5.2504) (103.9817, 5.5618) knots 0 0 0 1 2 2 2
  spline S129 degree 2 poles (103.9817, 5.5618) (103.8582, 5.8732) (103.4281, 6.1945) (103.087, 6.1945) knots 0 0 0 1 2 2 2
  spline S130 degree 2 poles (103.087, 6.1945) (102.7459, 6.1945) (102.306, 5.8732) (102.1775, 5.5519) knots 0 0 0 1 2 2 2
  spline S131 degree 2 poles (102.1775, 5.5519) (102.0539, 5.2405) (101.9649, 4.2914) (101.9649, 3.6932) knots 0 0 0 1 2 2 2
  spline S132 degree 2 poles (101.9649, 3.6932) (101.9649, 3.0506) (102.044, 2.1905) (102.1725, 1.8543) knots 0 0 0 1 2 2 2
  spline S133 degree 2 poles (102.1725, 1.8543) (102.2911, 1.538) (102.7311, 1.1969) (103.087, 1.1969) knots 0 0 0 1 2 2 2
  spline S134 degree 2 poles (103.087, 1.1969) (103.4232, 1.1969) (103.8631, 1.5182) (103.9867, 1.8395) knots 0 0 0 1 2 2 2
  line L202 (109.271, 0.6482) -> (106.2952, 0.6482)
  line L203 (106.2952, 0.6482) -> (106.2952, 1.271)
  line L204 (106.2952, 1.271) -> (107.4025, 1.271)
  line L205 (107.4025, 1.271) -> (107.4025, 5.3591)
  line L206 (107.4025, 5.3591) -> (106.2952, 5.3591)
  line L207 (106.2952, 5.3591) -> (106.2952, 5.9177)
  spline S135 degree 2 poles (106.2952, 5.9177) (106.923, 5.9177) (107.5162, 6.2736) (107.5557, 6.768) knots 0 0 0 1 2 2 2
  line L208 (107.5557, 6.768) -> (108.1885, 6.768)
  line L209 (108.1885, 6.768) -> (108.1885, 1.271)
  line L210 (108.1885, 1.271) -> (109.271, 1.271)
  line L211 (109.271, 1.271) -> (109.271, 0.6482)
  point P0 (140, 0)
  constraints: 4 other
extrude "돌출5" cut sketch "스케치4" against normal blind 2
sketch "스케치6" plane through (-170, -140, 0) normal (-1, 0, 0) x (0, 0, 1)
  line L0 (70, 85) -> (10, 85)
  line L1 (10, 85) -> (10, 25)
  line L2 (10, 25) -> (70, 25)
  line L3 (70, 25) -> (70, 85)
  line L4 (0, 0) -> (150, 0) projected
  line L5 (0, 110) -> (150, 110) projected
  line L6 (0, 110) -> (0, 0) projected
  circle A0 centre (65, 80) radius 2.15
  circle A1 centre (65, 30) radius 2.15
  circle A2 centre (15, 30) radius 2.15
  circle A3 centre (15, 80) radius 2.15
  circle A4 centre (40, 55) radius 27.5
  line L7 (67.5, 55) -> (12.5, 55)
  line L8 (40, 27.5) -> (40, 82.5)
  line L9 (42.5, 27.5) -> (42.5, 82.5)
  line L10 (37.5, 27.6139) -> (37.5, 82.5)
  line L11 (67.5, 52.5) -> (12.5, 52.5)
  line L12 (67.5, 57.5) -> (12.5, 57.5)
  line L13 (40, 52.5) -> (37.5, 52.5)
  line L14 (37.5, 52.5) -> (37.5, 25.6764)
  line L15 (37.5, 25.6764) -> (40, 25.6764)
  line L16 (40, 25.6764) -> (40, 52.5)
  line L17 (40, 55) -> (59.4454, 74.4454)
  line L18 (40, 55) -> (67.5, 55) construction
  line L19 (40, 55) -> (20.5546, 35.5546)
  line L20 (40, 55) -> (59.4454, 35.5546)
  line L21 (40, 55) -> (20.5546, 74.4454)
  line L22 (39.2929, 55.7071) -> (58.7383, 75.1525)
  line L23 (40.7071, 54.2929) -> (60.1525, 73.7383)
  line L24 (40.7071, 55.7071) -> (60.1525, 36.2617)
  line L25 (39.2929, 54.2929) -> (58.7383, 34.8475)
  line L26 (40.7071, 54.2929) -> (21.2617, 34.8475)
  line L27 (39.2929, 55.7071) -> (19.8475, 36.2617)
  line L28 (40.7071, 55.7071) -> (21.2617, 75.1525)
  line L29 (39.2929, 54.2929) -> (19.8475, 73.7383)
  point P0 (0, 140)
  point P1 (40, 85)
  point P2 (12.6139, 52.5)
  point P3 (67.3861, 52.5)
  point P4 (42.5, 52.5)
  point P5 (42.5, 27.6139)
  point P6 (42.5, 57.5)
  point P7 (67.3861, 57.5)
  point P8 (42.5, 82.3861)
  point P9 (12.6139, 57.5)
  point P10 (37.5, 57.5)
  point P11 (37.5, 82.3861)
  point P12 (37.5, 27.6139)
  point P13 (37.5, 51.0858)
  point P14 (21.2745, 34.8603)
  point P15 (19.8603, 36.2745)
  point P16 (36.0858, 52.5)
  point P17 (36.0858, 57.5)
  point P18 (19.8603, 73.7255)
  point P19 (21.2745, 75.1397)
  point P20 (37.5, 58.9142)
  point P21 (42.5, 58.9142)
  point P22 (58.7255, 75.1397)
  point P23 (60.1397, 73.7255)
  point P24 (43.9142, 57.5)
  point P25 (43.9142, 52.5)
  point P26 (60.1397, 36.2745)
  point P27 (58.7255, 34.8603)
  point P28 (42.5, 51.0858)
  dimension "d63" = 55
  dimension "d44" = 60
  dimension "d45" = 60
  dimension "d46" = 110
  dimension "d47" = 25
  dimension "d50" = 10
  dimension "d51" = 4.3
  dimension "d52" = 4.3
  dimension "d53" = 4.3
  dimension "d54" = 4.3
  dimension "d55" = 50
  dimension "d56" = 50
  dimension "d57" = 50
  dimension "d58" = 50
  dimension "d59" = 50
  dimension "d60" = 50
  dimension "d61" = 5
  dimension "d62" = 5
  dimension "d81" = 2.5
  dimension "d82" = 2.5
  dimension "d83" = 2.5
  dimension "d84" = 2.5
  dimension "d85" = 45
  dimension "d86" = 1
  dimension "d87" = 1
  dimension "d88" = 1
  dimension "d89" = 1
  dimension "d90" = 1
  dimension "d91" = 1
  dimension "d92" = 1
  dimension "d93" = 1
  constraints: 54 end point, 16 parallel, 4 centre point, 4 perpendicular, 3 horizontal, 2 midpoint, 2 point on line, 1 equal length, 11 other
  measures "d44" distance of L2.end L1.end
  measures "d45" distance of L1.end L0.end
  measures "d46" distance between parallel lines of L4 L5
  measures "d47" distance from line of L5 point (40, 85)
  measures "d50" distance between parallel lines of L6 L1
  measures "d51" diameter of A0
  measures "d52" diameter of A1
  measures "d53" diameter of A2
  measures "d54" diameter of A3
  measures "d55" distance of A3.centre A0.centre
  measures "d56" horizontal distance of A2.centre A0.centre
  measures "d57" distance of A2.centre A3.centre
  measures "d58" distance of A1.centre A2.centre
  measures "d59" distance of A1.centre A0.centre
  measures "d60" horizontal distance of A1.centre A3.centre
  measures "d61" distance from line of L0 A0.centre
  measures "d62" distance from line of L1 A3.centre
  measures "d81" distance between parallel lines of L8 L9
  measures "d82" distance between parallel lines of L8 L10
  measures "d83" distance between parallel lines of L7 L11
  measures "d84" distance between parallel lines of L7 L12
  measures "d85" angle of L18 L17
  measures "d86" distance between parallel lines of L17 L22
  measures "d87" distance between parallel lines of L17 L23
  measures "d88" distance between parallel lines of L20 L24
  measures "d89" distance between parallel lines of L20 L25
  measures "d90" distance between parallel lines of L19 L26
  measures "d91" distance between parallel lines of L19 L27
  measures "d92" distance between parallel lines of L21 L28
  measures "d93" distance between parallel lines of L21 L29
extrude "돌출6" cut sketch "스케치6" against normal blind 245 contours A0 | A1 | A2 | A3 | A4 L26 L10 | L9 L25 A4 | A4 L11 L27 | L24 L11 A4 | A4 L29 L12 | L23 A4 L12 | L9 A4 L22 | L28 A4 L10
sketch "스케치7" plane through (0, -140, 0) normal (1, 0, 0) x (0, 0, -1)
  line L0 (-130, 110) -> (-130, 0) projected
  circle A0 centre (-130, 55) radius 5
  circle A1 centre (-130, 70) radius 5
  circle A2 centre (-130, 85) radius 5
  circle A3 centre (-130, 40) radius 5
  circle A4 centre (-130, 25) radius 5
  circle A5 centre (-130, 10) radius 5
  circle A6 centre (-130, 100) radius 5
  point P0 (0, 140)
  dimension "d66" = 10
  dimension "d67" = 10
  dimension "d68" = 10
  dimension "d69" = 10
  dimension "d70" = 10
  dimension "d71" = 15
  dimension "d72" = 15
  dimension "d73" = 15
  dimension "d74" = 15
  dimension "d75" = 10
  dimension "d76" = 10
  dimension "d77" = 15
  dimension "d78" = 15
  constraints: 7 centre point, 8 other
  measures "d66" diameter of A0
  measures "d67" diameter of A1
  measures "d68" diameter of A2
  measures "d69" diameter of A3
  measures "d70" diameter of A4
  measures "d71" distance of A0.centre A3.centre
  measures "d72" distance of A4.centre A3.centre
  measures "d73" distance of A1.centre A0.centre
  measures "d74" distance of A2.centre A1.centre
  measures "d75" diameter of A5
  measures "d76" diameter of A6
  measures "d77" distance of A4.centre A5.centre
  measures "d78" distance of A6.centre A2.centre
extrude "돌출7" cut sketch "스케치7" against normal blind 245
sketch "스케치8" plane through (-140, -170, 0) normal (0, -1, 0) x (1, 0, 0)
  line L0 (43, 73.5) -> (67, 73.5)
  line L1 (70, 70.5) -> (70, 43)
  line L2 (67, 40) -> (43, 40)
  line L3 (40, 43) -> (40, 70.5)
  circle A0 centre (37.05, 56.75) radius 1.65
  circle A1 centre (72.95, 56.75) radius 1.65
  arc A2 (43, 73.5) -> (40, 70.5) centre (43, 70.5) ccw
  arc A3 (70, 70.5) -> (67, 73.5) centre (67, 70.5) ccw
  arc A4 (67, 40) -> (70, 43) centre (67, 43) ccw
  arc A5 (40, 43) -> (43, 40) centre (43, 43) ccw
  line L4 (0, 0) -> (0, 150) projected
  line L5 (110, 0) -> (110, 150) projected
  line L6 (0, 0) -> (110, 0) projected
  point P0 (140, 0)
  point P1 (70, 40)
  point P2 (70, 73.5)
  point P3 (40, 40)
  point P4 (40, 56.75)
  point P5 (70, 56.75)
  point P6 (55, 0)
  dimension "d94" = 30
  dimension "d95" = 33.5
  dimension "d96" = 3.3
  dimension "d97" = 3.3
  dimension "d98" = 16.75
  dimension "d99" = 16.75
  dimension "d100" = 35.9
  dimension "d101" = 2.95
  dimension "d102" = 2.95
  dimension "d103" = 3
  dimension "d104" = 40
  dimension "d105" = 40
  dimension "d106" = 40
  constraints: 8 end point, 8 point on circle, 8 tangent, 6 centre point, 6 point on line, 3 equal radius, 3 midpoint, 2 parallel, 1 horizontal, 1 perpendicular
  measures "d94" distance of point (70, 40) point (40, 40)
  measures "d95" distance of point (70, 73.5) point (70, 40)
  measures "d96" diameter of A0
  measures "d97" diameter of A1
  measures "d98" distance from line of L2 A0.centre
  measures "d99" distance from line of L0 A1.centre
  measures "d100" distance of A1.centre A0.centre
  measures "d101" distance of point (40, 56.75) A0.centre
  measures "d102" distance of point (70, 56.75) A1.centre
  measures "d103" radius of A2
  measures "d104" distance between parallel lines of L4 L3
  measures "d105" distance between parallel lines of L5 L1
  measures "d106" distance from line of point (55, 0) L2
extrude "돌출8" cut sketch "스케치8" against normal blind 5
